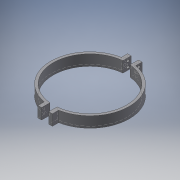
# Autodesk Inventor part: bottle clamp
Saved by Autodesk Inventor 2019 (Build 230136000, 136)
## iProperties
Created: 2022-03-28
Part Number: bottle clamp
Material: Generic
Document SubType Name: Modeling
Designer: Ian
Density: 1 g/cm^3
Appearance: Default
Author: Ian
Autodesk Inventor part; units mm, degrees
ref_plane "YZ Plane" through (0, 0, 0) normal (1, 0, 0) x (0, 1, 0)
ref_plane "XZ Plane" through (0, 0, 0) normal (0, 1, 0) x (-1, 0, 0)
ref_plane "XY Plane" through (0, 0, 0) normal (0, 0, 1) x (1, 0, 0)
sketch "Sketch1" plane through (0, 0, 0) normal (0, 1, 0) x (-1, 0, 0)
  circle A0 centre (-65.7542, 44.2448) radius 50.8 projected
  circle A1 centre (-65.7542, 44.2448) radius 50.9
  line L0 (-65.7542, 98.6448) -> (-65.7542, -10.1552)
  line L1 (-70.7542, 98.4145) -> (-70.7542, 94.8986)
  line L2 (-70.7542, -6.4091) -> (-70.7542, -9.925)
  line L3 (-60.7542, 98.4145) -> (-60.7542, 94.8986)
  line L4 (-60.7542, -6.4091) -> (-60.7542, -9.925)
  line L5 (-60.7542, 98.4145) -> (-60.7542, 106.4145)
  line L6 (-60.7542, 106.4145) -> (-55.7542, 106.4145)
  line L7 (-55.7542, 106.4145) -> (-55.7542, 97.7178)
  line L8 (-70.7542, 98.4145) -> (-70.7542, 106.4145)
  line L9 (-70.7542, 106.4145) -> (-75.7542, 106.4145)
  line L10 (-75.7542, 106.4145) -> (-75.7542, 97.7178)
  arc A2 (-60.7542, 98.4145) -> (-70.7542, 98.4145) centre (-65.7542, 44.2448) ccw
  line L11 (-70.7542, -9.925) -> (-70.7542, -17.925)
  line L12 (-70.7542, -17.925) -> (-75.7542, -17.925)
  line L13 (-75.7542, -17.925) -> (-75.7542, -9.2282)
  line L14 (-60.7542, -9.925) -> (-60.7542, -17.925)
  line L15 (-60.7542, -17.925) -> (-55.7542, -17.925)
  line L16 (-55.7542, -17.925) -> (-55.7542, -9.2282)
  arc A3 (-55.7542, -9.2282) -> (-55.7542, 97.7178) centre (-65.7542, 44.2448) ccw
  arc A4 (-75.7542, 97.7178) -> (-75.7542, -9.2282) centre (-65.7542, 44.2448) ccw
  arc A5 (-70.7542, -9.925) -> (-60.7542, -9.925) centre (-65.7542, 44.2448) ccw
  point P0 (0, 0)
  dimension "d0" = 0.1
  dimension "d4" = 5
  dimension "d5" = 5
  dimension "d6" = 5
  dimension "d7" = 5
  dimension "d10" = 8
  dimension "d11" = 5
  dimension "d12" = 8
  dimension "d13" = 5
  dimension "d15" = 3.5
  dimension "d16" = 8
  dimension "d17" = 5
  dimension "d18" = 8
  dimension "d19" = 5
  constraints: 34 end point, 14 point on circle, 6 perpendicular, 5 centre point, 4 line through centre, 4 parallel, 4 point on line, 3 vertical
  measures "d0" radial gap between concentric circles of A0 A1
  measures "d4" distance between parallel lines of L0 L1
  measures "d5" distance between parallel lines of L3 L0
  measures "d6" distance between parallel lines of L2 L0
  measures "d7" distance between parallel lines of L0 L4
  measures "d10" distance of L3.start L5.end
  measures "d11" distance of L5.end L6.end
  measures "d12" distance of L1.start L8.end
  measures "d13" distance of L8.end L9.end
  measures "d15" radial gap between concentric circles of A2 A1
  measures "d16" distance of L2.end L11.end
  measures "d17" distance of L11.end L12.end
  measures "d18" distance of L4.end L14.end
  measures "d19" distance of L14.end L15.end
extrude "Extrusion1" add sketch "Sketch1" along normal blind 15 contours L3 L5 L6 L7 A3 L16 L15 L14 L4 A1 | A1 L2 L11 L12 L13 A4 L10 L9 L8 L1
sketch "Sketch2" plane through (75.7542, 0, 106.4145) normal (1, 0, 0) x (0, 0, -1)
  circle A0 centre (119.9911, 11.25) radius 1.75
  circle A1 centre (119.9911, 3.75) radius 1.75
  circle A2 centre (119.9911, 3.75) radius 3.5
  circle A3 centre (119.9911, 11.25) radius 3.5
  line L0 (115.6427, 15) -> (124.3395, 15) projected
  line L1 (119.9911, 15) -> (119.9911, 11.25)
  line L2 (119.9911, 11.25) -> (119.9911, 7.5)
  line L3 (119.9911, 7.5) -> (119.9911, 3.75)
  line L4 (119.9911, 3.75) -> (119.9911, 0)
  line L5 (124.3395, 0) -> (112.8236, 0) projected
  point P0 (106.4145, 0)
  dimension "d20" = 3.5
  dimension "d21" = 3.5
  dimension "d22" = 7
  dimension "d23" = 7
  constraints: 8 end point, 4 centre point, 4 collinear, 2 coincident, 2 point on line, 2 vertical, 1 midpoint
  measures "d20" diameter of A0
  measures "d21" diameter of A1
  measures "d22" diameter of A2
  measures "d23" diameter of A3
extrude "Extrusion2" cut sketch "Sketch2" against normal through all contours A0 L2 L1 | L1 L2 A0 | L3 L4 A1 | A1 L4 L3
body "Solid1"
